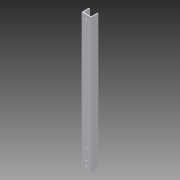
# Autodesk Inventor part: 18in C-Channel Rear
Saved by Autodesk Inventor 2013 (Build 170138000, 138)
## iProperties
Created: 2013-01-08
Part Number: 18in C-Channel Rear
Material: Aluminum 6061
Document SubType Name: Modeling
Designer: Naphat
Density: 1 g/cm^3
Author: Naphat
Autodesk Inventor part; units mm, degrees
ref_plane "YZ Plane" through (0, 0, 0) normal (1, 0, 0) x (0, 1, 0)
ref_plane "XZ Plane" through (0, 0, 0) normal (0, 1, 0) x (-1, 0, 0)
ref_plane "XY Plane" through (0, 0, 0) normal (0, 0, 1) x (1, 0, 0)
sketch "Sketch1" plane through (0, 0, 0) normal (0, 0, 1) x (1, 0, 0)
  line L0 (-16, 12.5) -> (-13, 12.5)
  line L1 (-13, 12.5) -> (-13, -9.5)
  line L2 (-13, -9.5) -> (13, -9.5)
  line L3 (13, -9.5) -> (13, 12.5)
  line L4 (13, 12.5) -> (16, 12.5)
  line L5 (16, 12.5) -> (16, -12.5)
  line L6 (16, -12.5) -> (-16, -12.5)
  line L7 (-16, -12.5) -> (-16, 12.5)
  point P0 (0, 0)
  dimension "d0" = 3
  dimension "d2" = 3
  dimension "d3" = 25
  dimension "d4" = 32
  dimension "d5" = 16
  dimension "d7" = 12.5
  dimension "d8" = 3
  dimension "d38" = 25
  constraints: 16 end point, 5 parallel, 1 collinear, 1 horizontal, 1 perpendicular
  measures "d0" distance of L0.start L0.end
  measures "d2" distance of L3.end L4.end
  measures "d3" distance of L6.end L0.start
  measures "d4" distance of L5.end L6.end
  measures "d5" distance from line of point (0, 0) L7
  measures "d7" distance from line of L6 point (0, 0)
  measures "d8" distance between parallel lines of L6 L2
  measures "d38" distance between parallel lines of L6 L4
extrude "Extrusion1" add sketch "Sketch1" against normal blind 457.2
sketch "Sketch6" plane through (-16, -12.5, 0) normal (0, -1, 0) x (1, 0, 0)
  circle A0 centre (16, -444.7) radius 3.175
  line L0 (32, -457.2) -> (0, -457.2) projected
  line L1 (32, 0) -> (32, -457.2) projected
  line L2 (32, 0) -> (0, 0) projected
  circle A1 centre (16, -12.5) radius 3.175
  line L3 (0, 0) -> (0, -457.2) projected
  line L4 (32, -435.2) -> (0, -435.2) construction
  line L5 (32, -385.2) -> (0, -385.2) construction
  line L6 (32, -388.2) -> (0, -388.2) construction
  circle A2 centre (16, -394.55) radius 3.175
  circle A3 centre (16, -428.85) radius 3.175
  point P0 (16, 0)
  dimension "d21" = 6.35
  dimension "d36" = 16
  dimension "d37" = 12.5
  dimension "d39" = 6.35
  dimension "d40" = 12.5
  dimension "d57" = 22
  dimension "d58" = 50
  dimension "d59" = 3
  dimension "d61" = 6.35
  dimension "d62" = 6.35
  dimension "d63" = 6.35
  constraints: 6 end point, 6 point on line, 4 centre point, 3 perpendicular, 3 vertical alignment, 1 equal radius
  measures "d21" diameter of A0
  measures "d36" distance from line of A0.centre L1
  measures "d37" distance from line of A0.centre L0
  measures "d39" diameter of A1
  measures "d40" distance from line of L2 A1.centre
  measures "d57" distance between parallel lines of L0 L4
  measures "d58" distance between parallel lines of L5 L4
  measures "d59" distance between parallel lines of L5 L6
  measures "d61" diameter of A2
  measures "d62" distance from line of L6 A2.centre
  measures "d63" distance from line of L4 A3.centre
hole "Hole1" at (0, -12.5, -12.5) at (0, -12.5, -444.7) at (0, -12.5, -394.55) at (0, -12.5, -428.85) direction (0, 1, 0) diameter 6.35 depth 3 tip angle 118
equation "\"d2\" = d0"
equation "\"d5\" = 0.5 * d4"
equation "\"d7\" = 0.5 * d3"
equation "\"d8\" = d0"
equation "\"d40\" = d37"
equation "\"d63\" = d62"
body "Solid1"
